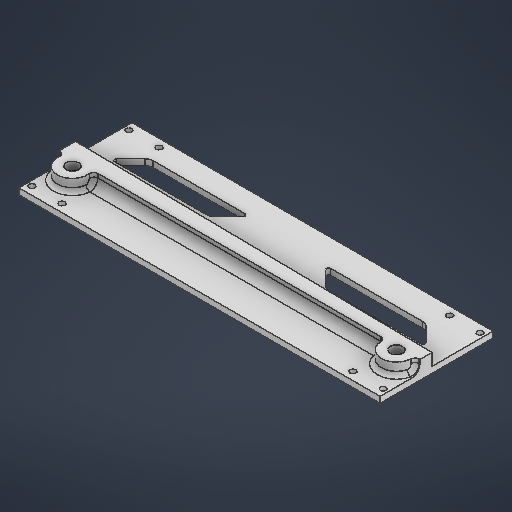
# Autodesk Inventor part: rigid_support1
Saved by Autodesk Inventor 2026.1 (Build 301233000, 233)
## iProperties
Created: 2025-10-27
Part Number: rigid_support1
Material: Generic
Document SubType Name: Modeling
Designer: emanuel
Density: 1 g/cm^3
Appearance: Default
Author: emanuel
Autodesk Inventor part; units mm, degrees
ref_plane "YZ Plane" through (0, 0, 0) normal (1, 0, 0) x (0, 1, 0)
ref_plane "XZ Plane" through (0, 0, 0) normal (0, 1, 0) x (-1, 0, 0)
ref_plane "XY Plane" through (0, 0, 0) normal (0, 0, 1) x (1, 0, 0)
sketch "Sketch1" plane through (0, 0, 0) normal (0, 1, 0) x (-1, 0, 0)
  line L0 (0, 0) -> (15, 0)
  line L1 (15, 0) -> (15, -48.3)
  line L2 (15, -48.3) -> (0, -48.3)
  line L3 (0, -48.3) -> (0, 0)
  circle A0 centre (15, 0) radius 1.5
  circle A1 centre (0, 0) radius 1.5
  circle A2 centre (15, -48.3) radius 1.5
  circle A3 centre (0, -48.3) radius 1.5
  line L4 (15, 0) -> (17.5, 0)
  line L5 (17.5, 0) -> (17.5, 4)
  line L6 (17.5, 4) -> (15, 4)
  line L7 (15, 4) -> (15, 0)
  line L8 (0, -48.3) -> (-2.5, -48.3)
  line L9 (-2.5, -48.3) -> (-2.5, -52.3)
  line L10 (-2.5, -52.3) -> (0, -52.3)
  line L11 (0, -52.3) -> (0, -48.3)
  line L12 (-2.5, -52.3) -> (17.5, -52.3)
  line L13 (17.5, -52.3) -> (17.5, 4)
  line L14 (17.5, 4) -> (-2.5, 4)
  line L15 (-2.5, 4) -> (-2.5, -52.3)
  line L16 (17.5, 4) -> (-47.5, 4)
  line L17 (-47.5, 4) -> (-47.5, -26)
  line L18 (-47.5, -26) -> (17.5, -26)
  line L19 (17.5, -26) -> (17.5, 4)
  circle A4 centre (-47.5, -26) radius 1.5
  line L20 (17.5, 4) -> (-72.5, 4)
  line L21 (17.5, 4) -> (-72.5, 4)
  line L22 (-72.5, 4) -> (-72.5, -44.8)
  line L23 (-72.5, -44.8) -> (17.5, -44.8)
  line L24 (17.5, -44.8) -> (17.5, 4)
  line L25 (-47.5, -26) -> (-57.5, -26)
  line L26 (-57.5, -26) -> (-67.5, -26)
  circle A5 centre (-67.5, -26) radius 1.5
  circle A6 centre (-57.5, -26) radius 1.5
  line L27 (-2.5, -52.3) -> (-72.5, -52.3)
  line L28 (-72.5, -52.3) -> (-72.5, -44.8)
  line L29 (-72.5, -44.8) -> (-2.5, -44.8)
  line L30 (-2.5, -44.8) -> (-2.5, -52.3)
  line L31 (-145, 0) -> (-160, 0)
  line L32 (-160, 0) -> (-160, -48.3)
  line L33 (-160, -48.3) -> (-145, -48.3)
  line L34 (-145, -48.3) -> (-145, 0)
  circle A7 centre (-160, 0) radius 1.5
  circle A8 centre (-145, 0) radius 1.5
  circle A9 centre (-160, -48.3) radius 1.5
  circle A10 centre (-145, -48.3) radius 1.5
  line L35 (-160, 0) -> (-162.5, 0)
  line L36 (-162.5, 0) -> (-162.5, 4)
  line L37 (-162.5, 4) -> (-160, 4)
  line L38 (-160, 4) -> (-160, 0)
  line L39 (-145, -48.3) -> (-142.5, -48.3)
  line L40 (-142.5, -48.3) -> (-142.5, -52.3)
  line L41 (-142.5, -52.3) -> (-145, -52.3)
  line L42 (-145, -52.3) -> (-145, -48.3)
  line L43 (-142.5, -52.3) -> (-162.5, -52.3)
  line L44 (-162.5, -52.3) -> (-162.5, 4)
  line L45 (-162.5, 4) -> (-142.5, 4)
  line L46 (-142.5, 4) -> (-142.5, -52.3)
  line L47 (-162.5, 4) -> (-97.5, 4)
  line L48 (-97.5, 4) -> (-97.5, -26)
  line L49 (-97.5, -26) -> (-162.5, -26)
  line L50 (-162.5, -26) -> (-162.5, 4)
  circle A11 centre (-97.5, -26) radius 1.5
  line L51 (-162.5, 4) -> (-72.5, 4)
  line L52 (-162.5, 4) -> (-72.5, 4)
  line L53 (-72.5, -44.8) -> (-162.5, -44.8)
  line L54 (-162.5, -44.8) -> (-162.5, 4)
  line L55 (-97.5, -26) -> (-87.5, -26)
  line L56 (-87.5, -26) -> (-77.5, -26)
  circle A12 centre (-77.5, -26) radius 1.5
  circle A13 centre (-87.5, -26) radius 1.5
  line L57 (-142.5, -52.3) -> (-72.5, -52.3)
  line L58 (-72.5, -44.8) -> (-142.5, -44.8)
  line L59 (-142.5, -44.8) -> (-142.5, -52.3)
  point P0 (0, -52.3)
  point P1 (-2.5, -46.3)
  point P2 (16.5, 0)
  point P3 (15, 1.5)
  dimension "d0" = 15
  dimension "d1" = 48.3
  dimension "d2" = 3
  dimension "d3" = 3
  dimension "d4" = 3
  dimension "d5" = 3
  dimension "d6" = 2.5
  dimension "d7" = 4
  dimension "d8" = 2.5
  dimension "d9" = 4
  dimension "d12" = 3
  dimension "d14" = 10
  dimension "d15" = 10
  dimension "d18" = 3
  dimension "d19" = 3
  dimension "d53" = 30
  constraints: 120 end point, 26 symmetric about line, 14 centre point, 14 coincident, 14 parallel, 8 horizontal, 8 perpendicular, 2 point on line, 7 other
  measures "d0" distance of L1.end L2.end
  measures "d1" distance of L0.end L1.end
  measures "d2" diameter of A0
  measures "d3" diameter of A1
  measures "d4" diameter of A2
  measures "d5" diameter of A3
  measures "d6" distance of L6.end L5.end
  measures "d7" distance of L5.end L4.end
  measures "d8" distance of L10.end L9.end
  measures "d9" distance of L9.end L8.end
  measures "d12" diameter of A4
  measures "d14" distance of L25.start L25.end
  measures "d15" distance of L25.end L26.end
  measures "d18" diameter of A5
  measures "d19" diameter of A6
  measures "d53" distance of L16.end L17.end
extrude "Extrusion1" add sketch "Sketch1" along normal blind 3 contours A1 L3 L18 L15 L14 L7 A0 L0 | L0 A0 L1 L18 L3 A1 | L18 L1 L23 L3 | L3 L23 L15 L18 | L7 L6 L5 L4 A0 | A0 L4 L13 L18 L1 | L23 L1 A2 L2 A3 L3 | L3 A3 L8 L15 L23 | L18 A4 L17 L16 L15 | L15 L23 L22 L20 L17 A4 L18 | L18 L13 L23 L1 | L15 L9 L27 L28 L23 | L23 L13 L12 L11 A3 L2 A2 L1 | A3 L11 L10 L9 L8 | L53 L46 L49 A11 L48 L51 L22 | L28 L57 L40 L46 L53 | L53 L34 L49 L46 | L46 L39 A10 L34 L53 | L48 A11 L49 L46 L47 | L41 L42 A10 L39 L40 | L49 L34 A8 L31 A7 L38 L45 L46 | L53 L32 L49 L34 | L34 A10 L33 A9 L32 L53 | L43 L44 L53 L32 A9 L33 A10 L42 | L49 L32 A7 L31 A8 L34 | L53 L44 L49 L32 | L38 A7 L35 L36 L37 | L49 L44 L35 A7 L32
sketch "Sketch2" plane through (0, 3, 0) normal (0, 1, 0) x (1, 0, 0)
  line L0 (-17.5, 52.3) -> (-17.5, -4) projected
  line L1 (-17.5, 24.15) -> (162.5, 21.9)
  line L2 (162.5, -2.5) -> (162.5, 46.3) projected
  line L3 (162.5, 21.9) -> (-17.5, 21.9)
  line L4 (-17.5, 21.9) -> (-17.5, 15.9)
  line L5 (-17.5, 15.9) -> (162.5, 15.9)
  line L6 (162.5, 15.9) -> (162.5, 21.9)
  line L7 (-17.5, -4) -> (-7.5, -4)
  line L8 (-7.5, -4) -> (-7.5, 12.65)
  line L9 (-7.5, 12.65) -> (-17.5, 12.65)
  line L10 (-17.5, 12.65) -> (-17.5, -4)
  circle A0 centre (-7.5, 12.65) radius 3.1
  circle A1 centre (-7.5, 12.65) radius 7.5
  line L11 (-17.5, -2.5) -> (162.5, -2.5) projected
  line L12 (162.5, -2.5) -> (152.5, -2.5)
  line L13 (152.5, -2.5) -> (152.5, 14.15)
  line L14 (152.5, 14.15) -> (162.5, 14.15)
  line L15 (162.5, 14.15) -> (162.5, -2.5)
  circle A2 centre (152.5, 14.15) radius 3.1
  circle A3 centre (152.5, 14.15) radius 7.5
  point P0 (0, 0)
  point P1 (-0.7407, 15.9)
  point P2 (145.207, 15.9)
  point P3 (159.793, 15.9)
  point P4 (-14.2593, 15.9)
  dimension "d24" = 6
  dimension "d44" = 10
  dimension "d45" = 16.65
  dimension "d46" = 6.2
  dimension "d47" = 10
  dimension "d48" = 16.65
  dimension "d49" = 6.2
  dimension "d50" = 15
  constraints: 26 end point, 6 parallel, 4 centre point, 4 coincident, 3 horizontal, 3 perpendicular, 2 midpoint, 1 point on line, 1 other
  measures "d24" distance of L4.end L3.end
  measures "d44" distance of L9.end L8.end
  measures "d45" distance of L8.end L7.end
  measures "d46" diameter of A0
  measures "d47" distance of L13.end L14.end
  measures "d48" distance of L12.end L13.end
  measures "d49" diameter of A2
  measures "d50" diameter of A3
extrude "Extrusion2" add sketch "Sketch2" along normal blind 6 contours L1 L3 L0 | L3 L2 L5 A3 A1 L0 | A1 L5 | L5 A1 L8 A0 L9 | A3 L14 A2 L5 | L5 A2 A3 | L9 A0 L8 A1 | A3 L13 A2 L14 | L5 A2 L13 A3
fillet "Fillet1" radius 4 3 edges at (72.2331, 3, -15.9) (-15.8796, 3, -15.9) (161.1465, 3, -15.9)
sketch "Sketch3" plane through (0, 3, 0) normal (0, 1, 0) x (1, 0, 0)
  line L0 (162.5, 21.9) -> (-17.5, 24.15) projected
  line L1 (162.5, 21.9) -> (122.5, 21.9)
  line L2 (122.5, 21.9) -> (122.5, 33.9)
  line L3 (122.5, 33.9) -> (162.5, 33.9)
  line L4 (162.5, 33.9) -> (162.5, 21.9)
  line L5 (-17.5, 52.3) -> (-17.5, 24.15) projected
  line L6 (-17.5, 24.15) -> (22.5, 24.15)
  line L7 (22.5, 24.15) -> (22.5, 36.15)
  line L8 (22.5, 36.15) -> (-17.5, 36.15)
  line L9 (-17.5, 36.15) -> (-17.5, 24.15)
  line L10 (142.5, 28.9) -> (102.5, 28.9)
  line L11 (102.5, 28.9) -> (102.5, 38.9)
  line L12 (102.5, 38.9) -> (142.5, 38.9)
  line L13 (142.5, 38.9) -> (142.5, 28.9)
  line L14 (142.5, 28.9) -> (102.5, 38.9) construction
  line L15 (102.5, 28.9) -> (142.5, 38.9) construction
  line L16 (42.5, 41.15) -> (2.5, 41.15)
  line L17 (2.5, 41.15) -> (2.5, 31.15)
  line L18 (2.5, 31.15) -> (42.5, 31.15)
  line L19 (42.5, 31.15) -> (42.5, 41.15)
  line L20 (42.5, 41.15) -> (2.5, 31.15) construction
  line L21 (2.5, 41.15) -> (42.5, 31.15) construction
  line L22 (142.5, 28.9) -> (152.5, 28.9)
  line L23 (152.5, 28.9) -> (142.5, 38.9)
  line L24 (102.5, 38.9) -> (92.5, 38.9)
  line L25 (92.5, 38.9) -> (102.5, 28.9)
  line L26 (42.5, 41.15) -> (52.5, 41.15)
  line L27 (52.5, 41.15) -> (42.5, 31.15)
  line L28 (2.5, 31.15) -> (-7.5, 31.15)
  line L29 (-7.5, 31.15) -> (2.5, 41.15)
  line L30 (42.5, 31.15) -> (2.5, 31.15)
  line L31 (2.5, 31.15) -> (2.5, 41.15)
  line L32 (2.5, 41.15) -> (42.5, 41.15)
  line L33 (42.5, 41.15) -> (42.5, 31.15)
  line L34 (142.5, 28.9) -> (102.5, 28.9)
  line L35 (102.5, 28.9) -> (102.5, 38.9)
  line L36 (102.5, 38.9) -> (142.5, 38.9)
  line L37 (142.5, 38.9) -> (142.5, 28.9)
  point P0 (0, 0)
  dimension "d28" = 40
  dimension "d29" = 12
  dimension "d30" = 40
  dimension "d31" = 12
  dimension "d32" = 40
  dimension "d33" = 10
  dimension "d34" = 40
  dimension "d35" = 10
  dimension "d36" = 10
  dimension "d37" = 10
  dimension "d38" = 10
  dimension "d39" = 10
  constraints: 72 end point, 15 parallel, 8 horizontal, 6 perpendicular, 4 midpoint, 3 point on line
  measures "d28" distance of L2.end L3.end
  measures "d29" distance of L1.end L2.end
  measures "d30" distance of L8.end L7.end
  measures "d31" distance of L7.end L6.end
  measures "d32" distance of L11.end L12.end
  measures "d33" distance of L10.end L11.end
  measures "d34" distance of L18.end L17.end
  measures "d35" distance of L17.end L16.end
  measures "d36" distance of L10.start L22.end
  measures "d37" distance of L11.end L24.end
  measures "d38" distance of L16.start L26.end
  measures "d39" distance of L17.end L28.end
extrude "Extrusion3" cut sketch "Sketch3" against normal blind 6 contours L10 L11 L12 L13 L3 L2 | L2 L3 L13 L10 | L23 L22 L13 L3 | L3 L13 L23 | L25 L24 L11 | L29 L17 L8 | L8 L17 L28 L29 | L17 L16 L19 L18 L7 L8 | L8 L7 L18 L17 | L26 L27 L19
fillet "Fillet2" radius 1 4 edges at (152.5, 1.5, -28.9) (92.5, 1.5, -38.9) (52.5, 1.5, -41.15) (-7.5, 1.5, -31.15)
fillet "Fillet3" radius 4 4 edges at (142.5, 1.5, -38.9) (102.5, 1.5, -28.9) (42.5, 1.5, -31.15) (2.5, 1.5, -41.15)
fillet "Fillet4" radius 2 10 edges at (-0.7407, 8, -15.9) (-7.5, 3, -5.15) (-14.6421, 4.3992, -14.9391) (-14.2593, 8, -15.9) (-0.3579, 4.3993, -14.9391) (145.0402, 4.3829, -14.925) (145.207, 8, -15.9) (159.9598, 4.3836, -14.9257) (159.793, 8, -15.9) (152.5, 3, -6.65)
body "Solid1"
